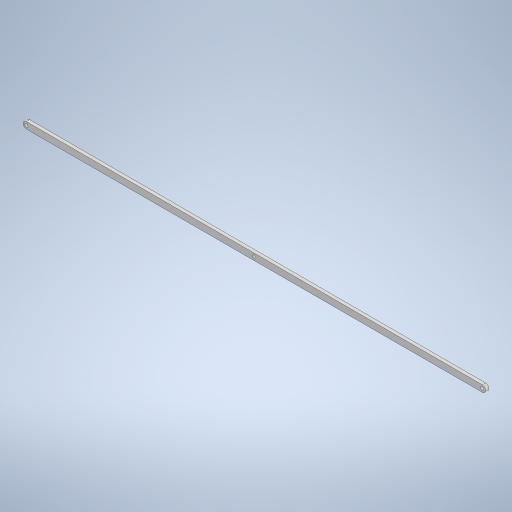
# Autodesk Inventor part: 5
Saved by Autodesk Inventor 2024 (Build 280153000, 153)
## iProperties
Created: 2025-09-18
Part Number: 5
Material: Generic
Document SubType Name: Modeling
Designer: Hello
Density: 1 g/cm^3
Appearance: Default
Mass: 280.785 g
Surface Area: 857.279 cm^2
Volume: 280.785 cm^3
Author: Hello
Autodesk Inventor part; units mm, degrees
ref_plane "YZ Plane" through (0, 0, 0) normal (1, 0, 0) x (0, 1, 0)
ref_plane "XZ Plane" through (0, 0, 0) normal (0, 1, 0) x (-1, 0, 0)
ref_plane "XY Plane" through (0, 0, 0) normal (0, 0, 1) x (1, 0, 0)
sketch "Sketch1" plane through (0, 0, 0) normal (0, 0, 1) x (1, 0, 0)
  circle A0 centre (0, 0) radius 5
  arc A1 (0, 10) -> (0, -10) centre (0, 0) ccw
  line L0 (0, 0) -> (200, 0)
  circle A2 centre (1400, 0) radius 5
  arc A3 (1400, -10) -> (1400, 10) centre (1400, 0) ccw
  line L1 (0, 10) -> (1400, 10)
  line L2 (0, -10) -> (1400, -10)
  dimension "d0" = 10
  dimension "d1" = 20
  dimension "d3" = 10
  dimension "d4" = 20
  dimension "d7" = 1400
  constraints: 6 end point, 4 centre point, 4 point on circle, 3 coincident, 2 tangent, 1 horizontal
  measures "d0" diameter of A0
  measures "d1" diameter of A1
  measures "d3" diameter of A2
  measures "d4" diameter of A3
  measures "d7" distance of A2.centre A0.centre
extrude "Extrusion1" add sketch "Sketch1" along normal blind 10
sketch "Sketch3" plane through (0, 0, 10) normal (0, 0, 1) x (1, 0, 0)
  circle A0 centre (700, 0) radius 5
  point P0 (0, 0)
  dimension "d8" = 10
  dimension "d11" = 700
  constraints: 1 centre point
  measures "d8" diameter of A0
  measures "d11" distance of A0.centre point (0, 0)
extrude "Extrusion2" cut sketch "Sketch3" against normal blind 10
body "Solid1"
